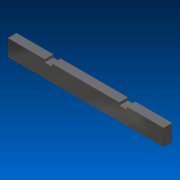
# Autodesk Inventor part: BB FRONT A SPACER 1
Saved by Autodesk Inventor 2012 (Build 160160000, 160)
## iProperties
Created: 2012-07-05
Part Number: BB FRONT A SPACER 1
Material: Default
Document SubType Name: Modeling
Designer: Hemant
Density: 1 g/cm^3
Author: Hemant
Autodesk Inventor part; units mm, degrees
ref_plane "YZ Plane" through (0, 0, 0) normal (1, 0, 0) x (0, 1, 0)
ref_plane "XZ Plane" through (0, 0, 0) normal (0, 1, 0) x (-1, 0, 0)
ref_plane "XY Plane" through (0, 0, 0) normal (0, 0, 1) x (1, 0, 0)
sketch "Sketch1" plane through (0, 0, 0) normal (0, 0, 1) x (1, 0, 0)
  line L0 (0, 0) -> (0, 58.2168)
  line L1 (0, 58.2168) -> (129.54, 58.2168)
  line L2 (129.54, 58.2168) -> (129.54, 48.6918)
  line L3 (129.54, 48.6918) -> (154.94, 48.6918)
  line L4 (154.94, 48.6918) -> (154.94, 58.2168)
  line L5 (154.94, 58.2168) -> (391.16, 58.2168)
  line L6 (391.16, 58.2168) -> (391.16, 48.6918)
  line L7 (391.16, 48.6918) -> (416.56, 48.6918)
  line L8 (416.56, 48.6918) -> (416.56, 58.2168)
  line L9 (416.56, 58.2168) -> (546.1, 58.2168)
  line L10 (546.1, 58.2168) -> (546.1, 0)
  line L11 (546.1, 0) -> (0, 0)
  dimension "d0" = 9.525
  dimension "d1" = 58.2168
  dimension "d2" = 546.1
  dimension "d3" = 129.54
  dimension "d4" = 129.54
  dimension "d5" = 25.4
  dimension "d6" = 25.4
  constraints: 24 end point, 8 parallel, 5 collinear, 1 perpendicular, 1 vertical
  measures "d0" distance between parallel lines of L3 L1
  measures "d1" distance between parallel lines of L1 L11
  measures "d2" distance between parallel lines of L10 L0
  measures "d3" distance between parallel lines of L2 L0
  measures "d4" distance between parallel lines of L10 L8
  measures "d5" distance between parallel lines of L8 L6
  measures "d6" distance between parallel lines of L4 L2
extrude "Extrusion1" add sketch "Sketch1" along normal blind 30.48
body "Solid1"
